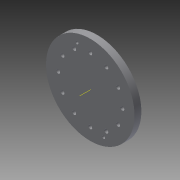
# Autodesk Inventor part: bay container 12 bottom
Saved by Autodesk Inventor 2015 (Build 190159000, 159)
## iProperties
Created: 2014-10-01
Part Number: bay container 12 bottom
Material: Generic
Document SubType Name: Modeling
Designer: ericd_000
Density: 1 g/cm^3
Appearance: Default
Author: ericd_000
Autodesk Inventor part; units mm, degrees
ref_plane "YZ Plane" through (0, 0, 0) normal (1, 0, 0) x (0, 1, 0)
ref_plane "XZ Plane" through (0, 0, 0) normal (0, 1, 0) x (-1, 0, 0)
ref_plane "XY Plane" through (0, 0, 0) normal (0, 0, 1) x (1, 0, 0)
sketch "Sketch1" plane through (0, 0, 0) normal (0, 1, 0) x (-1, 0, 0)
  circle A0 centre (0, 0) radius 45.5
  dimension "d0" = 91
  constraints: 1 centre point, 1 coincident
  measures "d0" diameter of A0
extrude "Extrusion1" add sketch "Sketch1" along normal blind 7
sketch "Sketch5" plane through (0, 7, 0) normal (0, 1, 0) x (1, 0, 0)
  circle A0 centre (0, 0) radius 6
  dimension "d27" = 12
  constraints: 1 centre point, 1 coincident
  measures "d27" diameter of A0
extrude "Extrusion5" add sketch "Sketch5" along normal blind 2
sketch "Sketch7" plane through (0, 0, 0) normal (0, -1, 0) x (1, 0, 0)
  circle A0 centre (0, 0) radius 45.5 projected
  line L0 (0, 0) -> (33, 0)
  circle A1 centre (33, 0) radius 2
  dimension "d37" = 4
  dimension "d38" = 33
  constraints: 2 end point, 1 centre point, 1 coincident, 1 horizontal
  measures "d37" diameter of A1
  measures "d38" distance of L0.start L0.end
extrude "Extrusion7" cut sketch "Sketch7" against normal blind 10 contours A1
pattern_circular "Circular Pattern1" count 12 over 360 about axis through (0, 0, 0) along (0, -1, 0) of "Extrusion7"
sketch "Sketch8" plane through (0, 0, 0) normal (0, -1, 0) x (1, 0, 0)
  circle A0 centre (-13.726, 35.2198) radius 1.5
  circle A1 centre (13.726, -35.2198) radius 1.5
  circle A2 centre (-16.5, 28.5788) radius 2 projected
  line L0 (-13.726, 35.2198) -> (13.726, -35.2198) construction
  point P0 (0, 0)
  point P1 (0, 0)
  dimension "d46" = 3
  dimension "d48" = 3
  dimension "d51" = 6.641
  dimension "d52" = 75.6
  constraints: 2 centre point, 2 end point, 1 coincident, 1 midpoint
  measures "d46" diameter of A0
  measures "d48" diameter of A1
  measures "d51" vertical distance of L0.start A2.centre
  measures "d52" distance of L0.start L0.end
extrude "Extrusion8" cut sketch "Sketch8" against normal blind 10 contours A0 | A1
body "Solid1"
